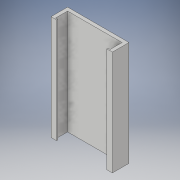
# Autodesk Inventor part: Phone Mount
Saved by Autodesk Inventor 2018 (Build 220112000, 112)
## iProperties
Created: 2018-08-14
Part Number: Phone Mount
Material: Generic
Document SubType Name: Modeling
Designer: F8PLTW
Density: 1 g/cm^3
Appearance: Default
Author: F8PLTW
Autodesk Inventor part; units mm, degrees
ref_plane "YZ Plane" through (0, 0, 0) normal (1, 0, 0) x (0, 1, 0)
ref_plane "XZ Plane" through (0, 0, 0) normal (0, 1, 0) x (-1, 0, 0)
ref_plane "XY Plane" through (0, 0, 0) normal (0, 0, 1) x (1, 0, 0)
sketch "Sketch1" plane through (0, 0, 0) normal (0, 0, 1) x (1, 0, 0)
  line L0 (-9.7052, 150.741) -> (79.6698, 150.741)
  line L1 (79.6698, 150.741) -> (79.6698, -1.659)
  line L2 (79.6698, -1.659) -> (-9.7052, -1.659)
  line L3 (-9.7052, -1.659) -> (-9.7052, 150.741)
  point P0 (0, 0)
  dimension "d0" = 89.375
  dimension "d1" = 152.4
  constraints: 8 end point, 2 parallel, 1 horizontal, 1 perpendicular
  measures "d0" distance of L1.end L2.end
  measures "d1" distance of L2.end L0.start
extrude "Extrusion1" add sketch "Sketch1" along normal blind 5.08
sketch "Sketch2" plane through (0, 0, 5.08) normal (0, 0, 1) x (1, 0, 0)
  line L0 (79.6698, 150.741) -> (-9.7052, 150.741) projected
  line L1 (-9.7052, -1.659) -> (79.6698, -1.659) projected
  line L2 (-9.7052, 150.741) -> (-4.7052, 150.741)
  line L3 (-4.7052, 150.741) -> (-4.7052, -1.659)
  line L4 (-4.7052, -1.659) -> (-9.7052, -1.659)
  line L5 (-9.7052, -1.659) -> (-9.7052, 150.741)
  line L6 (79.6698, 150.741) -> (74.6698, 150.741)
  line L7 (74.6698, 150.741) -> (74.6698, -1.659)
  line L8 (74.6698, -1.659) -> (79.6698, -1.659)
  line L9 (79.6698, -1.659) -> (79.6698, 150.741)
  point P0 (0, 0)
  dimension "d4" = 5
  dimension "d5" = 5
  constraints: 16 end point, 4 parallel, 2 horizontal, 2 perpendicular, 2 point on line
  measures "d4" distance of L3.end L4.end
  measures "d5" distance of L8.end L7.end
extrude "Extrusion2" add sketch "Sketch2" along normal blind 19.05 contours L9 L1 L7 L0 | L3 L1 L5 L0
sketch "Sketch3" plane through (-4.7052, -1.659, 5.08) normal (1, 0, 0) x (0, 0, -1)
  line L0 (0, 152.4) -> (-19.05, 152.4) projected
  line L1 (0, 0) -> (-19.05, 0) projected
  line L2 (-19.05, 152.4) -> (-17.4625, 152.4)
  line L3 (-17.4625, 152.4) -> (-17.4625, 0)
  line L4 (-17.4625, 0) -> (-19.05, 0)
  line L5 (-19.05, 0) -> (-19.05, 152.4)
  point P0 (5.08, 1.659)
  dimension "d8" = 1.5875
  constraints: 8 end point, 2 parallel, 1 horizontal, 1 perpendicular, 1 point on line
  measures "d8" distance of L3.end L4.end
sketch "Sketch4" plane through (74.6698, -1.659, 5.08) normal (-1, 0, 0) x (0, 0, 1)
  line L0 (19.05, 152.4) -> (19.05, 0) projected
  line L1 (0, 0) -> (19.05, 0) projected
  line L2 (19.05, 152.4) -> (17.4625, 152.4)
  line L3 (17.4625, 152.4) -> (17.4625, 0)
  line L4 (17.4625, 0) -> (19.05, 0)
  line L5 (19.05, 0) -> (19.05, 152.4)
  point P0 (-5.08, 1.659)
  dimension "d9" = 1.5875
  constraints: 8 end point, 2 parallel, 1 horizontal, 1 perpendicular, 1 point on line
  measures "d9" distance of L4.end L3.end
extrude "Extrusion3" add sketch "Sketch4" along normal blind 3.175
extrude "Extrusion4" add sketch "Sketch3" along normal blind 3.175
body "Solid1"
